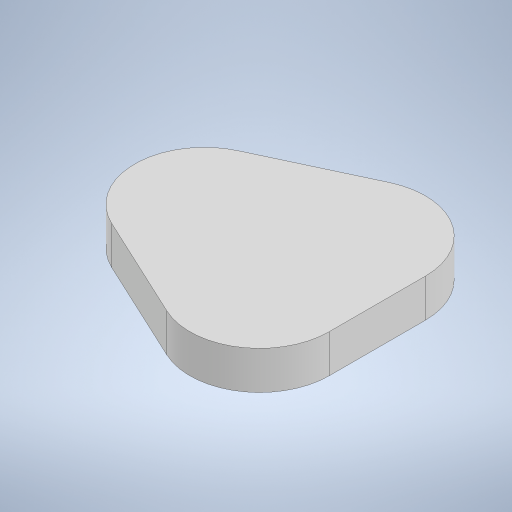
# Autodesk Inventor part: Tri_Box
Saved by Autodesk Inventor 2024.3 (Build 283343000, 343)
## iProperties
Created: 2025-06-26
Part Number: Tri_Box
Material: Generic
Document SubType Name: Modeling
Designer: 1
Density: 1 g/cm^3
Appearance: Default
Author: 1
Autodesk Inventor part; units mm, degrees
ref_plane "YZ Plane" through (0, 0, 0) normal (1, 0, 0) x (0, 1, 0)
ref_plane "XZ Plane" through (0, 0, 0) normal (0, 1, 0) x (-1, 0, 0)
ref_plane "XY Plane" through (0, 0, 0) normal (0, 0, 1) x (1, 0, 0)
sketch "Sketch1" plane through (0, 0, 0) normal (0, 1, 0) x (-1, 0, 0)
  line L0 (72.8792, 0) -> (-46.0667, 0) projected
  line L1 (48.7883, 0) -> (-20.6188, 32.3651)
  line L2 (-20.6188, 32.3651) -> (-20.6188, -32.3651)
  line L3 (-20.6188, -32.3651) -> (48.7883, 0)
  circle A0 centre (-7.2188, -11.3313) radius 13.4
  circle A1 centre (-7.2188, 11.3313) radius 13.4
  circle A2 centre (17.0812, 0) radius 13.4
  circle A3 centre (0, 0) radius 20.6188
  line L4 (52.8138, 0) -> (-29.0745, 0)
  line L5 (-23.6188, -37.0741) -> (-23.6188, 37.0741)
  line L6 (-23.6188, 37.0741) -> (55.8869, 0)
  line L7 (-23.6188, -37.0741) -> (55.8869, 0)
  circle A4 centre (-7.2188, 11.3313) radius 16.4
  circle A5 centre (-7.2188, -11.3313) radius 16.4
  circle A6 centre (17.0812, 0) radius 16.4
  point P0 (-1.5557, -23.4758)
  point P1 (-20.6188, -11.3313)
  point P2 (-20.6188, 11.3313)
  point P3 (-1.5557, 23.4758)
  point P4 (22.7443, 12.1445)
  point P5 (22.7443, -12.1445)
  point P6 (-0.2879, -26.1947)
  point P7 (24.0121, -14.8634)
  point P8 (24.0121, 14.8634)
  point P9 (-0.2879, 26.1947)
  point P10 (-23.6188, 11.3313)
  point P11 (-23.6188, -11.3313)
  dimension "d9" = 50
  dimension "d10" = 26.8
  dimension "d11" = 37.7
  dimension "d12" = 26.8
  dimension "d13" = 26.8
  dimension "d14" = 3
  dimension "d15" = 3
  constraints: 14 end point, 12 tangent, 7 centre point, 4 coincident, 2 parallel, 2 vertical, 1 point on line, 2 other
  measures "d9" angle of L3 L1
  measures "d10" diameter of A0
  measures "d11" distance from line of L2 A2.centre
  measures "d12" diameter of A2
  measures "d13" diameter of A1
  measures "d14" distance between parallel lines of L2 L5
  measures "d15" distance between parallel lines of L3 L7
extrude "Extrusion1" add sketch "Sketch1" along normal blind 9 contours A6 L1 A4 L6 | A6 L1 | L7 A5 L3 A6 | A6 L3 | A4 L1 | A6 L0 A2 L1 | A5 L3 | L3 A2 L0 A6 | L1 A1 L2 A4 | A5 L2 A0 L3 | A4 L2 L0 L5 | A4 L2 | L5 L0 L2 A5 | A5 L2
sketch "Sketch2" plane through (0, 9, 0) normal (0, 1, 0) x (1, 0, 0)
  line L0 (0.2879, 26.1947) -> (-24.0121, 14.8634) projected
  arc A0 (23.6188, 11.3313) -> (0.2879, 26.1947) centre (7.2188, 11.3313) ccw projected
  line L1 (23.6188, -11.3313) -> (23.6188, 11.3313) projected
  arc A1 (0.2879, -26.1947) -> (23.6188, -11.3313) centre (7.2188, -11.3313) ccw projected
  line L2 (-24.0121, -14.8634) -> (0.2879, -26.1947) projected
  arc A2 (-24.0121, 14.8634) -> (-24.0121, -14.8634) centre (-17.0812, 0) ccw projected
  arc A3 (20.6188, 11.3313) -> (1.5557, 23.4758) centre (7.2188, 11.3313) ccw projected
  line L3 (-22.7443, 12.1445) -> (1.5557, 23.4758) projected
  arc A4 (-22.7443, 12.1445) -> (-22.7443, -12.1445) centre (-17.0812, 0) ccw projected
  line L4 (1.5557, -23.4758) -> (-22.7443, -12.1445) projected
  arc A5 (1.5557, -23.4758) -> (20.6188, -11.3313) centre (7.2188, -11.3313) ccw projected
  line L5 (20.6188, 11.3313) -> (20.6188, -11.3313) projected
extrude "Extrusion2" add sketch "Sketch2" against normal blind 2 contours L5 A5 L4 A4 L3 A3
body "Solid1"
